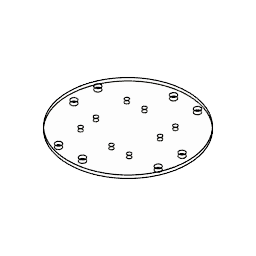
MidPlate_v4 (Autodesk Fusion 360 design; units mm, degrees)
Autodesk Fusion 360 part; units mm, degrees
derive "Sketch1" from "LowerPlate v12"
sketch "sketch 908" plane through (0, 0, 0) normal (0, 0, 1) x (1, 0, 0)
  circle A0 centre (0, 0) radius 60
  line L0 (-36.4192, 17.7153) -> (3.5808, 17.7153)
  line L1 (3.5808, 17.7153) -> (3.5808, -2.2847)
  line L2 (3.5808, -2.2847) -> (-36.4192, -2.2847)
  line L3 (-36.4192, -2.2847) -> (-36.4192, 17.7153)
  line L4 (-17.7153, -36.4192) -> (-17.7153, 3.5808)
  line L5 (-17.7153, 3.5808) -> (2.2847, 3.5808)
  line L6 (2.2847, 3.5808) -> (2.2847, -36.4192)
  line L7 (2.2847, -36.4192) -> (-17.7153, -36.4192)
  line L8 (36.4192, -17.7153) -> (-3.5808, -17.7153)
  line L9 (-3.5808, -17.7153) -> (-3.5808, 2.2847)
  line L10 (-3.5808, 2.2847) -> (36.4192, 2.2847)
  line L11 (36.4192, 2.2847) -> (36.4192, -17.7153)
  line L12 (17.7153, 36.4192) -> (17.7153, -3.5808)
  line L13 (17.7153, -3.5808) -> (-2.2847, -3.5808)
  line L14 (-2.2847, -3.5808) -> (-2.2847, 36.4192)
  line L15 (-2.2847, 36.4192) -> (17.7153, 36.4192)
  line L16 (-24.4192, 23.2153) -> (-24.4192, -7.7847) construction
  line L17 (-36.4192, 7.7153) -> (-24.4192, 7.7153) construction
  circle A1 centre (-24.4192, 23.2153) radius 2
  circle A2 centre (-24.4192, -7.7847) radius 2
  circle A3 centre (7.7847, -24.4192) radius 2
  circle A4 centre (-23.2153, -24.4192) radius 2
  circle A5 centre (24.4192, 7.7847) radius 2
  circle A6 centre (24.4192, -23.2153) radius 2
  circle A7 centre (-7.7847, 24.4192) radius 2
  circle A8 centre (23.2153, 24.4192) radius 2
  line L18 (-36.4192, 7.7153) -> (-50, 7.7153) construction
  line L19 (-50, 19.7153) -> (-50, -4.2847) construction
  circle A9 centre (-50, -4.2847) radius 3
  circle A10 centre (-50, 19.7153) radius 3
  circle A11 centre (-19.7153, -50) radius 3
  circle A12 centre (4.2847, -50) radius 3
  circle A13 centre (50, -19.7153) radius 3
  circle A14 centre (50, 4.2847) radius 3
  circle A15 centre (19.7153, 50) radius 3
  circle A16 centre (-4.2847, 50) radius 3
  point P0 (-24.4192, 7.7153)
extrude "Extrude2" add sketch "sketch 908" along normal blind 3 contours A0 | L0 L2 L3 L4 L5 L14 | L0 L1 L10 L12 L14 L15 | L0 L1 L5 L6 L10 L14 | L2 L4 L5 L9 L10 L14 | L5 L6 L10 L14 | L2 L4 L6 L7 L8 L9 | L1 L2 L6 L10 L12 L13 | L1 L2 L6 L10 | L2 L9 L10 L14 | L2 L6 L10 L14 | L2 L6 L8 L9 L13 L14 | L6 L8 L10 L11 L12 L13 | L2 L6 L13 L14
